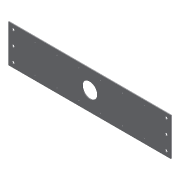
# Autodesk Inventor part: elevbackplt
Saved by Autodesk Inventor 2015 SP1 (Build 190203100, 203)
## iProperties
Created: 2015-01-20
Part Number: elevbackplt
Material: Generic
Document SubType Name: Modeling
Designer: Owner
Density: 1 g/cm^3
Appearance: Default
Author: Owner
Autodesk Inventor part; units mm, degrees
ref_plane "YZ Plane" through (0, 0, 0) normal (1, 0, 0) x (0, 1, 0)
ref_plane "XZ Plane" through (0, 0, 0) normal (0, 1, 0) x (-1, 0, 0)
ref_plane "XY Plane" through (0, 0, 0) normal (0, 0, 1) x (1, 0, 0)
sketch "Sketch1" plane through (0, 0, 0) normal (0, 0, 1) x (1, 0, 0)
  line L0 (0, 0) -> (436.118, 0)
  line L1 (436.118, 0) -> (436.118, 101.6)
  line L2 (436.118, 101.6) -> (0, 101.6)
  line L3 (0, 101.6) -> (0, 0)
  circle A0 centre (12.7, 88.9) radius 3.3655
  circle A1 centre (12.7, 50.8) radius 3.3655
  circle A2 centre (12.7, 12.7) radius 3.3655
  circle A3 centre (423.418, 88.9) radius 3.3655
  circle A4 centre (423.418, 50.8) radius 3.3655
  circle A5 centre (423.418, 12.7) radius 3.3655
  circle A6 centre (364.744, 12.7) radius 1.5875
  circle A7 centre (306.07, 12.7) radius 1.5875
  circle A8 centre (247.396, 12.7) radius 1.5875
  circle A9 centre (188.722, 12.7) radius 1.5875
  circle A10 centre (130.048, 12.7) radius 1.5875
  circle A11 centre (71.374, 12.7) radius 1.5875
  circle A12 centre (364.744, 88.9) radius 1.5875
  circle A13 centre (306.07, 88.9) radius 1.5875
  circle A14 centre (247.396, 88.9) radius 1.5875
  circle A15 centre (188.722, 88.9) radius 1.5875
  circle A16 centre (130.048, 88.9) radius 1.5875
  circle A17 centre (71.374, 88.9) radius 1.5875
  circle A18 centre (218.059, 50.8) radius 20.32
  dimension "d0" = 436.118
  dimension "d1" = 101.6
  dimension "d2" = 6.731
  dimension "d3" = 12.7
  dimension "d4" = 12.7
  dimension "d7" = 38.1
  dimension "d10" = 410.718
  dimension "d13" = 12.7
  dimension "d14" = 3.175
  dimension "d15" = 58.674
  dimension "d18" = 58.674
  dimension "d21" = 76.2
  dimension "d24" = 40.64
  dimension "d25" = 50.8
  dimension "d26" = 218.059
  constraints: 19 centre point, 8 end point, 3 horizontal, 2 parallel, 2 vertical, 1 perpendicular, 32 other
  measures "d0" distance of L2.end L1.end
  measures "d1" distance between parallel lines of L0 L2
  measures "d2" diameter of A0
  measures "d3" distance from line of L3 A0.centre
  measures "d4" distance from line of L2 A0.centre
  measures "d7" distance of A0.centre A1.centre
  measures "d10" distance of A0.centre A3.centre
  measures "d13" distance from line of A3.centre L1
  measures "d14" diameter of A6
  measures "d15" distance of A6.centre A5.centre
  measures "d18" distance of A6.centre A7.centre
  measures "d21" distance of A6.centre A12.centre
  measures "d24" diameter of A18
  measures "d25" distance from line of L2 A18.centre
  measures "d26" distance from line of L3 A18.centre
extrude "Extrusion1" add sketch "Sketch1" along normal blind 2.286
equation "\"d15\" = 0.142857 * d10"
equation "\"d26\" = 0.5 * d0"
body "Solid1"
